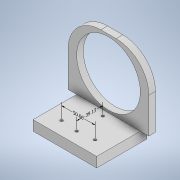
# Autodesk Inventor part: Harmonic Drive Mount
Saved by Autodesk Inventor 2022 (Build 260153000, 153)
## iProperties
Created: 2022-01-01
Part Number: Harmonic Drive Mount
Material: Generic
Document SubType Name: Modeling
Designer: Mlees
Density: 1 g/cm^3
Appearance: Default
Author: Mlees
Autodesk Inventor part; units mm, degrees
ref_plane "YZ Plane" through (0, 0, 0) normal (1, 0, 0) x (0, 1, 0)
ref_plane "XZ Plane" through (0, 0, 0) normal (0, 1, 0) x (-1, 0, 0)
ref_plane "XY Plane" through (0, 0, 0) normal (0, 0, 1) x (1, 0, 0)
sketch "Sketch1" plane through (0, 0, 0) normal (0, 1, 0) x (-1, 0, 0)
  line L0 (0, 0) -> (-94.996, 0)
  line L1 (-94.996, 0) -> (-94.996, -75)
  line L2 (-94.996, -75) -> (0, -75)
  line L3 (0, -75) -> (0, 0)
  dimension "d0" = 94.996
  dimension "d1" = 75
  constraints: 8 end point, 2 parallel, 1 horizontal, 1 perpendicular
  measures "d0" distance of L2.end L1.end
  measures "d1" distance of L1.end L0.end
extrude "Extrusion1" add sketch "Sketch1" along normal blind 15
sketch "Sketch2" plane through (0, 15, 0) normal (0, 1, 0) x (1, 0, 0)
  line L0 (94.996, 75) -> (0, 75) projected
  line L1 (0, 75) -> (-12.7, 75)
  line L2 (94.996, 0) -> (94.996, 75) projected
  line L3 (94.996, 75) -> (107.696, 75)
  line L4 (107.696, 75) -> (107.696, 65.094)
  line L5 (107.696, 65.094) -> (-12.7, 65.094)
  line L6 (-12.7, 65.094) -> (-12.7, 75)
  line L7 (0, 75) -> (94.996, 75)
  point P0 (0, 0)
  dimension "d4" = 12.7
  dimension "d5" = 12.7
  dimension "d6" = 9.906
  constraints: 12 end point, 2 horizontal, 2 perpendicular, 1 collinear, 1 vertical
  measures "d4" distance of L0.end L1.end
  measures "d5" distance of L0.start L3.end
  measures "d6" distance of L3.end L4.end
extrude "Extrusion2" add sketch "Sketch2" along normal blind 101.6
sketch "Sketch4" plane through (0, 0, 0) normal (0, -1, 0) x (1, 0, 0)
  line L0 (0, 0) -> (94.996, 0) projected
  line L1 (94.996, -75) -> (0, -75) projected
  circle A0 centre (47.498, -17.5525) radius 2
  circle A1 centre (47.498, -56.6788) radius 2
  dimension "d12" = 4
  dimension "d13" = 4
  constraints: 2 centre point
  measures "d12" diameter of A0
  measures "d13" diameter of A1
extrude "Extrusion4" cut sketch "Sketch4" against normal through all
sketch "Sketch5" plane through (-12.7, 15, -65.094) normal (0, 0, 1) x (1, 0, 0)
  line L0 (58.198, 0) -> (62.198, 0) projected
  line L1 (120.396, 0) -> (120.396, 101.6) projected
  circle A0 centre (60.198, 50.8) radius 47.5
  point P0 (12.7, -15)
  dimension "d17" = 95
  constraints: 1 centre point
  measures "d17" diameter of A0
extrude "Extrusion5" cut sketch "Sketch5" against normal through all
sketch "Sketch6" plane through (0, 15, 0) normal (0, 1, 0) x (1, 0, 0)
  line L0 (0, 0) -> (94.996, 0) projected
  circle A0 centre (72.498, 20) radius 2
  circle A1 centre (22.498, 20) radius 2
  dimension "d23" = 4
  constraints: 2 centre point
  measures "d23" diameter of A0
extrude "Extrusion6" cut sketch "Sketch6" against normal through all
chamfer "Chamfer1" distance 2 angle 45 2 edges at (70.498, 0, -20) (20.498, 0, -20)
fillet "Fillet1" radius 48.75 2 edges at (-12.7, 116.6, -70.047) (107.696, 116.6, -70.047)
body "Solid1"
